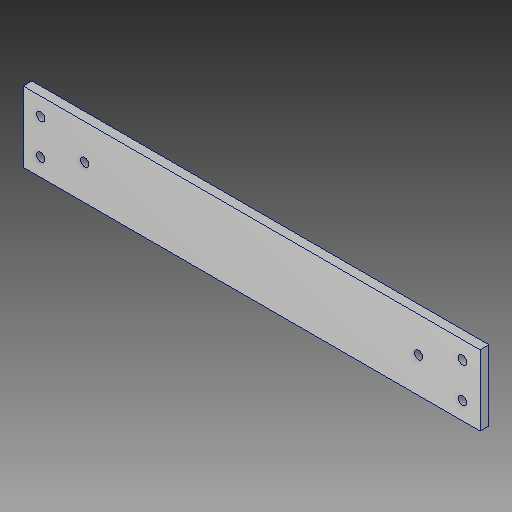
# Autodesk Inventor part: outbrace
Saved by Autodesk Inventor 2018.1 (Build 221171000, 171)
## iProperties
Created: 2017-08-13
Part Number: outbrace
Material: Aluminum 6061
Document SubType Name: Modeling
Designer: Kai
Density: 2.7 g/cm^3
Appearance: Aluminum - Flat
Author: Kai
Autodesk Inventor part; units mm, degrees
ref_plane "YZ Plane" through (0, 0, 0) normal (1, 0, 0) x (0, 1, 0)
ref_plane "XZ Plane" through (0, 0, 0) normal (0, 1, 0) x (-1, 0, 0)
ref_plane "XY Plane" through (0, 0, 0) normal (0, 0, 1) x (1, 0, 0)
sketch "Sketch1" plane through (0, 0, 0) normal (0, 0, 1) x (1, 0, 0)
  line L0 (0, 0) -> (-330.2, 0)
  line L1 (-330.2, 0) -> (-330.2, 50.8)
  line L2 (-330.2, 50.8) -> (0, 50.8)
  line L3 (0, 50.8) -> (0, 0)
  circle A0 centre (-12.7, 38.1) radius 3.1
  circle A1 centre (-12.7, 12.7) radius 3.1
  circle A2 centre (-317.5, 38.1) radius 3.1
  circle A3 centre (-317.5, 12.7) radius 3.1
  circle A4 centre (-285.75, 25.4) radius 3
  circle A5 centre (-44.45, 25.4) radius 3
  dimension "d0" = 330.2
  dimension "d1" = 50.8
  dimension "d2" = 6.2
  dimension "d3" = 6.2
  dimension "d4" = 6.2
  dimension "d5" = 6.2
  dimension "d6" = 12.7
  dimension "d7" = 12.7
  dimension "d8" = 25.4
  dimension "d9" = 12.7
  dimension "d10" = 12.7
  dimension "d11" = 12.7
  dimension "d12" = 25.4
  dimension "d13" = 12.7
  dimension "d16" = 6
  dimension "d17" = 44.45
  dimension "d18" = 6
  dimension "d19" = 44.45
  constraints: 8 end point, 6 centre point, 2 parallel, 1 horizontal, 1 perpendicular
  measures "d0" distance of L1.end L2.end
  measures "d1" distance of L0.end L1.end
  measures "d2" diameter of A0
  measures "d3" diameter of A1
  measures "d4" diameter of A2
  measures "d5" diameter of A3
  measures "d6" distance from line of L1 A2.centre
  measures "d7" distance from line of L1 A3.centre
  measures "d8" distance of A3.centre A2.centre
  measures "d9" distance from line of L2 A2.centre
  measures "d10" distance from line of L2 A0.centre
  measures "d11" distance from line of L3 A0.centre
  measures "d12" distance of A1.centre A0.centre
  measures "d13" distance from line of L3 A1.centre
  measures "d16" diameter of A4
  measures "d17" distance from line of L1 A4.centre
  measures "d18" diameter of A5
  measures "d19" distance from line of L3 A5.centre
extrude "Extrusion1" add sketch "Sketch1" along normal blind 6.35 contours L0 L1 L2 L3 | A4 | A5
sketch "Sketch2" plane through (0, 0, 6.35) normal (0, 0, 1) x (1, 0, 0)
  circle A0 centre (-44.45, 25.4) radius 3
  circle A1 centre (-285.75, 25.4) radius 3
  line L0 (0, 0) -> (0, 50.8) projected
  line L1 (-330.2, 50.8) -> (-330.2, 0) projected
  dimension "d20" = 6
  dimension "d21" = 6
  dimension "d22" = 44.45
  dimension "d23" = 44.45
  constraints: 2 centre point
  measures "d20" diameter of A0
  measures "d21" diameter of A1
  measures "d22" distance from line of L0 A0.centre
  measures "d23" distance from line of L1 A1.centre
extrude "Extrusion2" cut sketch "Sketch2" against normal blind 6.35
body "Solid1"
